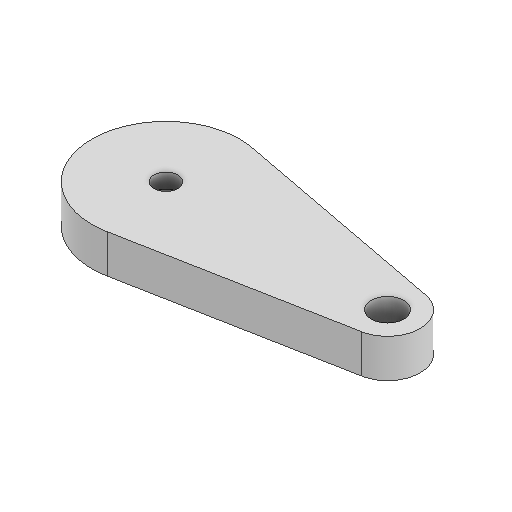
# Autodesk Inventor part: Servo Spinner
Saved by Autodesk Inventor 2025.1 (Build 291241020, 241B)
## iProperties
Created: 2024-12-02
Part Number: Servo Spinner
Material: Generic
Document SubType Name: Modeling
Designer: ALEXANDERNICHOLS
Density: 1 g/cm^3
Appearance: Default
Author: ALEXANDERNICHOLS
Autodesk Inventor part; units mm, degrees
ref_plane "YZ Plane" through (0, 0, 0) normal (1, 0, 0) x (0, 1, 0)
ref_plane "XZ Plane" through (0, 0, 0) normal (0, 1, 0) x (-1, 0, 0)
ref_plane "XY Plane" through (0, 0, 0) normal (0, 0, 1) x (1, 0, 0)
sketch "Sketch1" plane through (0, 0, 0) normal (0, 1, 0) x (-1, 0, 0)
  circle A0 centre (0, 0) radius 2.3368
  arc A1 (-1.1853, -6.2384) -> (-1.1853, 6.2384) centre (0, 0) ccw
  arc A2 (-19.5715, 2.7449) -> (-19.5715, -2.7449) centre (-19.05, 0) ccw
  line L0 (-1.1853, -6.2384) -> (-19.5715, -2.7449)
  line L1 (-19.5715, 2.7449) -> (-1.1853, 6.2384)
  circle A3 centre (-19.05, 0) radius 1.397
  arc A4 (-2.3333, -0.127) -> (-2.3333, 0.127) centre (-2.3368, 0) ccw
  arc A5 (-2.256, -0.6093) -> (-2.3088, -0.361) centre (-2.2857, -0.4858) ccw
  arc A6 (-2.08, -1.065) -> (-2.1833, -0.8331) centre (-2.1348, -0.9505) ccw
  arc A7 (-1.8131, -1.4742) -> (-1.9623, -1.2688) centre (-1.8905, -1.3735) ccw
  arc A8 (-1.467, -1.819) -> (-1.6557, -1.6491) centre (-1.5636, -1.7366) ccw
  arc A9 (-1.0567, -2.0842) -> (-1.2766, -1.9573) centre (-1.1684, -2.0237) ccw
  arc A10 (-0.6003, -2.2584) -> (-0.8418, -2.1799) centre (-0.7221, -2.2224) ccw
  arc A11 (-0.1176, -2.3338) -> (-0.3702, -2.3073) centre (-0.2443, -2.324) ccw
  arc A12 (0.3702, -2.3073) -> (0.1176, -2.3338) centre (0.2443, -2.324) ccw
  arc A13 (0.8418, -2.1799) -> (0.6003, -2.2584) centre (0.7221, -2.2224) ccw
  arc A14 (1.2766, -1.9573) -> (1.0567, -2.0842) centre (1.1684, -2.0237) ccw
  arc A15 (1.6557, -1.6491) -> (1.467, -1.819) centre (1.5636, -1.7366) ccw
  arc A16 (1.9623, -1.2688) -> (1.8131, -1.4742) centre (1.8905, -1.3735) ccw
  arc A17 (2.1833, -0.8331) -> (2.08, -1.065) centre (2.1348, -0.9505) ccw
  arc A18 (2.3088, -0.361) -> (2.256, -0.6093) centre (2.2857, -0.4858) ccw
  arc A19 (2.3333, 0.127) -> (2.3333, -0.127) centre (2.3368, 0) ccw
  arc A20 (2.256, 0.6093) -> (2.3088, 0.361) centre (2.2857, 0.4858) ccw
  arc A21 (2.08, 1.065) -> (2.1833, 0.8331) centre (2.1348, 0.9505) ccw
  arc A22 (1.8131, 1.4742) -> (1.9623, 1.2688) centre (1.8905, 1.3735) ccw
  arc A23 (1.467, 1.819) -> (1.6557, 1.6491) centre (1.5636, 1.7366) ccw
  arc A24 (1.0567, 2.0842) -> (1.2766, 1.9573) centre (1.1684, 2.0237) ccw
  arc A25 (0.6003, 2.2584) -> (0.8418, 2.1799) centre (0.7221, 2.2224) ccw
  arc A26 (0.1176, 2.3338) -> (0.3702, 2.3073) centre (0.2443, 2.324) ccw
  arc A27 (-0.3702, 2.3073) -> (-0.1176, 2.3338) centre (-0.2443, 2.324) ccw
  arc A28 (-0.8418, 2.1799) -> (-0.6003, 2.2584) centre (-0.7221, 2.2224) ccw
  arc A29 (-1.2766, 1.9573) -> (-1.0567, 2.0842) centre (-1.1684, 2.0237) ccw
  arc A30 (-1.6557, 1.6491) -> (-1.467, 1.819) centre (-1.5636, 1.7366) ccw
  arc A31 (-1.9623, 1.2688) -> (-1.8131, 1.4742) centre (-1.8905, 1.3735) ccw
  arc A32 (-2.1833, 0.8331) -> (-2.08, 1.065) centre (-2.1348, 0.9505) ccw
  arc A33 (-2.3088, 0.361) -> (-2.256, 0.6093) centre (-2.2857, 0.4858) ccw
  point P0 (-2.256, -0.6093)
  point P1 (-2.3088, -0.361)
  point P2 (-2.1833, -0.8331)
  point P3 (-1.8131, -1.4742)
  point P4 (-1.6557, -1.6491)
  point P5 (-1.0567, -2.0842)
  point P6 (-0.8418, -2.1799)
  point P7 (-0.1176, -2.3338)
  point P8 (-0.3702, -2.3073)
  point P9 (0.1176, -2.3338)
  point P10 (0.8418, -2.1799)
  point P11 (0.6003, -2.2584)
  point P12 (1.8131, -1.4742)
  point P13 (2.08, -1.065)
  point P14 (2.3088, -0.361)
  point P15 (2.256, -0.6093)
  point P16 (2.256, 0.6093)
  point P17 (2.3088, 0.361)
  point P18 (2.1833, 0.8331)
  point P19 (1.9623, 1.2688)
  point P20 (1.6557, 1.6491)
  point P21 (1.0567, 2.0842)
  point P22 (1.2766, 1.9573)
  point P23 (0.6003, 2.2584)
  point P24 (0.8418, 2.1799)
  point P25 (0.1176, 2.3338)
  point P26 (0.3702, 2.3073)
  point P27 (-0.1176, 2.3338)
  point P28 (-0.8418, 2.1799)
  point P29 (-0.6003, 2.2584)
  point P30 (-1.2766, 1.9573)
  point P31 (-1.0567, 2.0842)
  point P32 (-1.8131, 1.4742)
  point P33 (-2.08, 1.065)
  point P34 (-2.3088, 0.361)
  point P35 (-2.256, 0.6093)
  dimension "d0" = 4.6736
  dimension "d1" = 12.7
  dimension "d2" = 19.05
  dimension "d3" = 5.588
  dimension "d4" = 2.794
  dimension "d10" = 0.254
  dimension "d13" = 360
  constraints: 64 point on circle, 33 centre point, 4 end point, 4 tangent, 3 coincident, 1 horizontal alignment, 126 other
  measures "d1" diameter of A1
  measures "d2" distance of point (0, 0) A2.centre
  measures "d3" diameter of A2
  measures "d4" diameter of A3
  measures "d10" diameter of A4
extrude "Extrusion1" add sketch "Sketch1" along normal blind 2.032
sketch "Sketch2" plane through (0, 2.032, 0) normal (0, 1, 0) x (1, 0, 0)
  line L0 (19.5715, 2.7449) -> (1.1853, 6.2384) projected
  arc A0 (1.1853, 6.2384) -> (1.1853, -6.2384) centre (0, 0) ccw projected
  line L1 (1.1853, -6.2384) -> (19.5715, -2.7449) projected
  arc A1 (19.5715, -2.7449) -> (19.5715, 2.7449) centre (19.05, 0) ccw projected
  circle A2 centre (0, 0) radius 2.3368 projected
  circle A3 centre (19.05, 0) radius 1.397 projected
  circle A4 centre (0, 0) radius 1.016
  dimension "d7" = 2.032
  constraints: 1 centre point, 1 coincident
  measures "d7" diameter of A4
extrude "Extrusion2" add sketch "Sketch2" along normal blind 1.27 contours A1 L1 A0 L0 | A2
body "Solid1"
